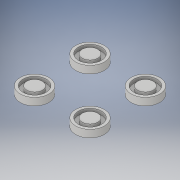
# Autodesk Inventor part: pé
Saved by Autodesk Inventor 2019.4 (Build 234330000, 330)
## iProperties
Created: 2019-10-19
Part Number: pé
Material: Genérico
Document SubType Name: Modeling
Designer: natha
Density: 1 g/cm^3
Appearance: Padrão
Author: natha
Autodesk Inventor part; units mm, degrees
ref_plane "YZ Plane" through (0, 0, 0) normal (1, 0, 0) x (0, 1, 0)
ref_plane "XZ Plane" through (0, 0, 0) normal (0, 1, 0) x (-1, 0, 0)
sketch "Esboço1" plane through (0, 0, 0) normal (0, 1, 0) x (-1, 0, 0)
  circle A0 centre (0, 0) radius 7.75
  line L0 (0, 0) -> (0, -30) construction
  circle A1 centre (0, -30) radius 7.75
  line L1 (0, -30) -> (0, -60) construction
  circle A2 centre (30, 0) radius 7.75
  line L2 (30, 0) -> (30, -30) construction
  circle A3 centre (30, -30) radius 7.75
  line L3 (30, -30) -> (30, -60) construction
  line L4 (0, 0) -> (30, 0) construction
  dimension "d0" = 15.5
  dimension "d1" = 30
  dimension "d2" = 15.5
  dimension "d3" = 30
  dimension "d4" = 15.5
  dimension "d5" = 30
  dimension "d6" = 15.5
  dimension "d7" = 30
  dimension "d8" = 30
  constraints: 10 end point, 4 centre point, 4 vertical, 1 coincident, 1 horizontal
  measures "d0" diameter of A0
  measures "d1" distance of L0.start L0.end
  measures "d2" diameter of A1
  measures "d3" distance of L1.start L1.end
  measures "d4" diameter of A2
  measures "d5" distance of L2.start L2.end
  measures "d6" diameter of A3
  measures "d7" distance of L3.start L3.end
  measures "d8" distance of L0.start L4.end
extrude "Extrusão1" add sketch "Esboço1" along normal blind 4
sketch "Esboço2" plane through (-30, 4, 0) normal (0, 1, 0) x (1, 0, 0)
  circle A0 centre (0, 0) radius 7.75 projected
  circle A1 centre (0, 30) radius 7.75 projected
  circle A2 centre (30, 30) radius 7.75 projected
  circle A3 centre (0, 0) radius 6.25
  circle A4 centre (0, 30) radius 6.25
  circle A5 centre (0, 0) radius 4.2
  circle A6 centre (0, 30) radius 4.2
  circle A7 centre (30, 0) radius 6.25
  circle A8 centre (30, 30) radius 6.25
  circle A9 centre (30, 0) radius 4.2
  circle A10 centre (30, 30) radius 4.2
  dimension "d12" = 12.5
  dimension "d13" = 12.5
  dimension "d17" = 8.4
  dimension "d18" = 8.4
  dimension "d25" = 12.5
  dimension "d26" = 12.5
  dimension "d27" = 8.4
  dimension "d28" = 8.4
  constraints: 8 centre point, 2 coincident
  measures "d12" diameter of A3
  measures "d13" diameter of A4
  measures "d17" diameter of A5
  measures "d18" diameter of A6
  measures "d25" diameter of A7
  measures "d26" diameter of A8
  measures "d27" diameter of A9
  measures "d28" diameter of A10
ref_plane "Plano de trabalho1" through (0, 1.5, 0) normal (0, 1, 0) x (1, 0, 0)
sketch "Esboço3" plane through (0, 1.5, 0) normal (0, 1, 0) x (1, 0, 0)
  circle A0 centre (0, 0) radius 2
  circle A1 centre (0, 30) radius 6.25 projected
  circle A2 centre (0, 30) radius 2
  dimension "d21" = 4
  dimension "d22" = 4
  constraints: 2 centre point, 2 coincident
  measures "d21" diameter of A0
  measures "d22" diameter of A2
extrude "Extrusão4" cut sketch "Esboço3" against normal blind 2.5 contours A0 | A2
extrude "Extrusão5" cut sketch "Esboço2" against normal blind 2 contours A3 | A4 | A7 | A8
